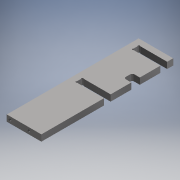
# Autodesk Inventor part: Rückhalter
Saved by Autodesk Inventor 2018 (Build 220112000, 112)
## iProperties
Created: 2013-03-04
Part Number: Rückhalter
Material: Stainless Steel
Document SubType Name: Modeling
Designer: Neef
Density: 8 g/cm^3
Appearance: Semi-Polished
Author: Neef
Autodesk Inventor part; units mm, degrees
ref_plane "YZ Plane" through (0, 0, 0) normal (1, 0, 0) x (0, 1, 0)
ref_plane "XZ Plane" through (0, 0, 0) normal (0, 1, 0) x (-1, 0, 0)
ref_plane "XY Plane" through (0, 0, 0) normal (0, 0, 1) x (1, 0, 0)
sketch "Skizze1" plane through (0, 0, 0) normal (0, 0, 1) x (1, 0, 0)
  line L0 (27.5, 0) -> (-27.5, 0)
  line L1 (-27.5, 0) -> (-27.5, 210)
  line L2 (-27.5, 210) -> (27.5, 210)
  line L3 (27.5, 210) -> (27.5, 0)
  line L4 (0, 252) -> (0, -42) projected
  line L5 (-38.5, 0) -> (38.5, 0) projected
  point P0 (0, 0)
  point P1 (0, 0)
  dimension "d0" = 210
  dimension "d1" = 55
  constraints: 8 end point, 2 parallel, 1 collinear, 1 horizontal, 1 midpoint, 1 perpendicular, 1 point on line
  measures "d0" distance of L2.end L0.start
  measures "d1" distance of L1.end L2.end
extrude "Extrusion1" add sketch "Skizze1" along normal blind 10
sketch "Skizze2" plane through (0, 0, 10) normal (0, 0, 1) x (1, 0, 0)
  line L0 (27.5, 210) -> (27.5, 0) projected
  circle A0 centre (3.5, 195.1) radius 4.3 projected
  circle A1 centre (-6.5, 192.1) radius 1.2295 projected
  circle A2 centre (-6.5, 198.1) radius 1.2295 projected
  line L1 (21.5, 200.1) -> (-17.5, 200.1) projected
  line L2 (-17.5, 190.1) -> (-17.5, 200.1) projected
  line L3 (21.5, 190.1) -> (-17.5, 190.1) projected
  line L4 (21.5, 190.1) -> (21.5, 200.1) projected
  line L5 (19.1583, 143.6) -> (26.6417, 143.6) projected
  arc A3 (19.1583, 156.6) -> (19.1583, 143.6) centre (22.9, 150.1) ccw projected
  line L6 (26.6417, 156.6) -> (19.1583, 156.6) projected
  arc A4 (26.6417, 143.6) -> (26.6417, 156.6) centre (22.9, 150.1) ccw projected
  circle A5 centre (3.5, 105.1) radius 4.3 projected
  circle A6 centre (-6.5, 102.1) radius 1.2295 projected
  circle A7 centre (-6.5, 108.1) radius 1.2295 projected
  line L7 (21.5, 110.1) -> (-17.5, 110.1) projected
  line L8 (-17.5, 100.1) -> (-17.5, 110.1) projected
  line L9 (21.5, 100.1) -> (-17.5, 100.1) projected
  line L10 (21.5, 100.1) -> (21.5, 110.1) projected
  line L11 (27.5, 200.4) -> (-15.4311, 200.4)
  line L12 (-15.4311, 189.8) -> (27.5, 189.8)
  line L13 (27.5, 189.8) -> (27.5, 200.4)
  arc A8 (-17.5, 191.8689) -> (-15.4311, 189.8) centre (-16.7, 190.6) ccw
  arc A9 (-15.4311, 200.4) -> (-17.5, 198.3311) centre (-16.7, 199.6) ccw
  line L14 (22.9, 150.1) -> (-7.7295, 150.1) construction
  line L15 (-17.5, 190.1) -> (-17.5, 189.8)
  line L16 (-17.5, 200.4) -> (-17.5, 200.1)
  line L17 (-17.5, 198.3311) -> (-17.5, 191.8689)
  circle A10 centre (3.5, 105.1) radius 4.3
  circle A11 centre (-6.5, 108.1) radius 1.2295
  circle A12 centre (-6.5, 102.1) radius 1.2295
  line L18 (21.5, 100.1) -> (-17.5, 100.1)
  line L19 (-17.5, 110.1) -> (-17.5, 100.1)
  line L20 (21.5, 110.1) -> (-17.5, 110.1)
  line L21 (21.5, 110.1) -> (21.5, 100.1)
  line L22 (27.5, 99.8) -> (-15.4311, 99.8)
  line L23 (-15.4311, 110.4) -> (27.5, 110.4)
  line L24 (27.5, 110.4) -> (27.5, 99.8)
  arc A13 (-15.4311, 110.4) -> (-17.5, 108.3311) centre (-16.7, 109.6) ccw
  arc A14 (-17.5, 101.8689) -> (-15.4311, 99.8) centre (-16.7, 100.6) ccw
  line L25 (-17.5, 110.1) -> (-17.5, 110.4)
  line L26 (-17.5, 99.8) -> (-17.5, 100.1)
  line L27 (-17.5, 101.8689) -> (-17.5, 108.3311)
  line L28 (27.5, 156.9) -> (18.4, 156.9)
  line L29 (15.4, 153.9) -> (15.4, 146.3)
  line L30 (18.4, 143.3) -> (27.5, 143.3)
  line L31 (27.5, 143.3) -> (27.5, 156.9)
  arc A15 (18.4, 156.9) -> (15.4, 153.9) centre (18.4, 153.9) ccw
  arc A16 (15.4, 146.3) -> (18.4, 143.3) centre (18.4, 146.3) ccw
  point P0 (0, 0)
  dimension "d4" = 0.3
  dimension "d5" = 0.3
  dimension "d6" = 3
  dimension "d7" = 3
  dimension "d8" = 0.8
  dimension "d9" = 0.8
  dimension "d10" = 0.8
  dimension "d11" = 0.8
  dimension "d13" = 10.6
  dimension "d15" = 0.3
  dimension "d16" = 0.3
  dimension "d17" = 12.1
  dimension "d18" = 3
  constraints: 38 end point, 13 symmetric about line, 12 point on circle, 6 centre point, 6 parallel, 6 point on line, 5 perpendicular, 4 tangent, 2 horizontal, 1 equal radius, 5 other
  measures "d4" distance between parallel lines of L11 L1
  measures "d5" distance between parallel lines of L3 L12
  measures "d6" diameter of A9
  measures "d7" diameter of A8
  measures "d8" distance from line of L11 A9.centre
  measures "d9" distance from line of L2 A9.centre
  measures "d10" distance from line of L12 A8.centre
  measures "d11" distance from line of L2 A8.centre
  measures "d13" distance of L16.start L15.end
  measures "d15" distance between parallel lines of L28 L6
  measures "d16" distance between parallel lines of L30 L5
  measures "d17" distance between parallel lines of L0 L29
  measures "d18" radius of A15
extrude "Extrusion2" cut sketch "Skizze2" against normal through all contours L0 L22 A14 L8 L9 L10 L7 A13 L23 | L0 A4 L6 A3 L29 A15 L28 | L0 L12 A8 L2 L3 L4 L1 A9 L11 | L2 L1 L4 L3 | A4 L0 | L0 A4 L5 A3 L6 | L0 L30 A16 L29 A3 L5 A4 | L8 L7 L10 L9 | A0 | A1 | A2 | A5 | A6 | A7
sketch "Skizze3" plane through (-27.5, 0, 0) normal (0, -1, 0) x (1, 0, 0)
  line L0 (55, 10) -> (0, 10) projected
  line L1 (0, 0) -> (0, 10) projected
  point P0 (27.5, 0)
  point P1 (5, 5)
  point P2 (35, 5)
  dimension "d21" = 30
  dimension "d22" = 5
  dimension "d23" = 5
  dimension "d24" = 5
  measures "d21" distance of point (5, 5) point (35, 5)
  measures "d22" distance from line of L1 point (5, 5)
  measures "d23" distance from line of L0 point (5, 5)
  measures "d24" distance from line of L0 point (35, 5)
hole "Bohrung1" at (-22.5, 0, 5) at (7.5, 0, 5) direction (0, 1, 0) diameter 4.134 depth 15 tip angle 118 thread size "M5x0.8" class "6H" standard "ISO Metric profile"
equation "\"d4\" = d5"
equation "\"d7\" = d6"
equation "\"d9\" = d8"
equation "\"d10\" = d8"
equation "\"d11\" = d10"
equation "\"d16\" = d15"
equation "\"d24\" = d23"
